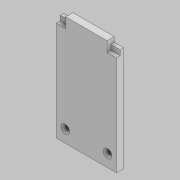
# Autodesk Inventor part: cover
Saved by Autodesk Inventor 2021.4 (Build 254397000, 397)
## iProperties
Created: 2022-11-07
Part Number: cover
Material: Generisch
Document SubType Name: Modeling
Designer: Tilman Preuschoff
Density: 1 g/cm^3
Appearance: Vorgabe
Author: Tilman Preuschoff
Autodesk Inventor part; units mm, degrees
ref_plane "YZ Plane" through (0, 0, 0) normal (1, 0, 0) x (0, 1, 0)
ref_plane "XZ Plane" through (0, 0, 0) normal (0, 1, 0) x (-1, 0, 0)
ref_plane "XY Plane" through (0, 0, 0) normal (0, 0, 1) x (1, 0, 0)
sketch "Skizze1" plane through (0, 0, 0) normal (0, 0, 1) x (1, 0, 0)
  line L0 (-12.5, 22.5) -> (12.5, 22.5)
  line L1 (12.5, 22.5) -> (12.5, -22.5)
  line L2 (12.5, -22.5) -> (-12.5, -22.5)
  line L3 (-12.5, -22.5) -> (-12.5, 22.5)
  line L4 (-12.5, 22.5) -> (12.5, -22.5) construction
  line L5 (12.5, 22.5) -> (-12.5, -22.5) construction
  point P0 (0, 0)
  dimension "d0" = 25
  dimension "d1" = 45
  constraints: 12 end point, 2 midpoint, 2 parallel, 1 horizontal, 1 perpendicular
  measures "d0" distance between parallel lines of L1 L3
  measures "d1" distance between parallel lines of L2 L0
extrude "Extrusion1" add sketch "Skizze1" along normal blind 3
sketch "Skizze8" plane through (-12.5, -22.5, 0) normal (0, -1, 0) x (1, 0, 0)
  line L0 (25, 0) -> (24.4, 0) projected
  line L1 (25, 3) -> (0, 3) projected
  line L2 (25, 0) -> (0, 0)
  line L3 (0, 0) -> (0, 3)
  line L4 (0, 3) -> (25, 3)
  line L5 (25, 3) -> (25, 0)
  point P0 (12.5, 0)
  constraints: 8 end point, 2 parallel, 1 horizontal, 1 perpendicular
extrude "Extrusion6" add sketch "Skizze8" along normal blind 0.7
sketch "Skizze9" plane through (0, 0, 3) normal (0, 0, 1) x (1, 0, 0)
  line L0 (12.5, 22.5) -> (-12.5, 22.5) projected
  line L1 (-12.5, 22.5) -> (-8.6, 22.5)
  line L2 (-8.6, 22.5) -> (-8.6, 20.4)
  line L3 (-8.6, 20.4) -> (-12.5, 20.4)
  line L4 (-12.5, 20.4) -> (-12.5, 22.5)
  line L5 (12.5, 22.5) -> (8.6, 22.5)
  line L6 (8.6, 22.5) -> (8.6, 20.4)
  line L7 (8.6, 20.4) -> (12.5, 20.4)
  line L8 (12.5, 20.4) -> (12.5, 22.5)
  point P0 (0, 0)
  dimension "d46" = 3.9
  dimension "d47" = 3.9
  dimension "d48" = 2.1
  dimension "d49" = 2.1
  constraints: 16 end point, 4 parallel, 2 horizontal, 2 perpendicular
  measures "d46" distance between parallel lines of L4 L2
  measures "d47" distance between parallel lines of L8 L6
  measures "d48" distance between parallel lines of L0 L3
  measures "d49" distance between parallel lines of L0 L7
extrude "Extrusion7" cut sketch "Skizze9" against normal through all
sketch "Skizze10" plane through (0, 0, 3) normal (0, 0, 1) x (1, 0, 0)
  line L0 (-8.8, -18.1) -> (8.8, -18.1)
  line L1 (-12.5, 20.4) -> (-12.5, -23.2) projected
  line L2 (12.5, 20.4) -> (12.5, -23.2) projected
  line L3 (12.5, -23.2) -> (-12.5, -23.2) projected
  point P0 (0, 0)
  dimension "d52" = 3.7
  dimension "d53" = 3.7
  dimension "d54" = 5.1
  constraints: 2 end point, 1 horizontal
  measures "d52" distance from line of L1 L0.start
  measures "d53" distance from line of L2 L0.end
  measures "d54" distance between parallel lines of L0 L3
hole "Bohrung2" at (8.8, -18.1, 3) at (-8.8, -18.1, 3) direction (0, 0, -1) diameter 1.8 depth 8 countersink diameter 3.6 countersink angle 90 clearance for "Flachkopfsenkschraube DIN EN ISO 2009" size "M1.6" standard "DIN"
sketch "Skizze11" plane through (0, 0, 3) normal (0, 0, 1) x (1, 0, 0)
  line L0 (-8.6, 20.4) -> (-12.5, 20.4)
  line L1 (-12.5, 20.4) -> (-12.5, 18.3)
  line L2 (-12.5, 18.3) -> (-8.6, 18.3)
  line L3 (-8.6, 18.3) -> (-8.6, 20.4)
  line L4 (8.6, 20.4) -> (12.5, 20.4) projected
  line L5 (8.6, 20.4) -> (12.5, 20.4)
  line L6 (12.5, 20.4) -> (12.5, 18.3)
  line L7 (12.5, 18.3) -> (8.6, 18.3)
  line L8 (8.6, 18.3) -> (8.6, 20.4)
  point P0 (0, 0)
  dimension "d62" = 2.1
  dimension "d63" = 2.1
  constraints: 16 end point, 4 parallel, 2 horizontal, 2 perpendicular, 2 vertical alignment
  measures "d62" distance between parallel lines of L0 L2
  measures "d63" distance between parallel lines of L4 L7
extrude "Extrusion8" cut sketch "Skizze11" against normal blind 1.55
